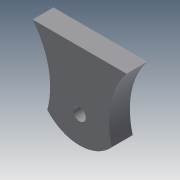
# Autodesk Inventor part: stojan1
Saved by Autodesk Inventor 2013 (Build 170138000, 138)
## iProperties
Created: 2013-05-11
Part Number: stojan1
Material: Generic
Document SubType Name: Modeling
Designer: idle-rug
Density: 1 g/cm^3
Author: idle-rug
Autodesk Inventor part; units mm, degrees
ref_plane "YZ Plane" through (0, 0, 0) normal (1, 0, 0) x (0, 1, 0)
ref_plane "XZ Plane" through (0, 0, 0) normal (0, 1, 0) x (-1, 0, 0)
ref_plane "XY Plane" through (0, 0, 0) normal (0, 0, 1) x (1, 0, 0)
sketch "Sketch1" plane through (0, 0, 0) normal (0, 1, 0) x (-1, 0, 0)
  circle A0 centre (0, 0) radius 3
  line L0 (-22.5, 28) -> (22.5, 28)
  line L1 (0, -13) -> (0, 28)
  arc A1 (22.5, 28) -> (15.4587, -5.964) centre (52.0868, 4.1543) ccw
  arc A2 (-15.4587, -5.964) -> (-22.5, 28) centre (-52.0868, 4.1543) ccw
  arc A3 (-15.4587, -5.964) -> (15.4587, -5.964) centre (0, 7.5) ccw
  dimension "d0" = 6
  dimension "d1" = 38
  dimension "d2" = 38
  dimension "d3" = 41
  dimension "d4" = 45
  constraints: 6 point on circle, 4 centre point, 4 end point, 1 coincident, 1 midpoint
  measures "d0" diameter of A0
  measures "d1" radius of A1
  measures "d2" radius of A2
  measures "d3" distance of L1.end L1.start
  measures "d4" distance of L0.start L0.end
extrude "Extrusion1" add sketch "Sketch1" along normal blind 10 contours A0 L1 L0 A1 A3 | A0 L1 A3 A2 L0
body "Solid1"
